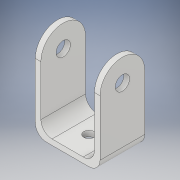
# Autodesk Inventor part: MainMount
Saved by Autodesk Inventor 2018 (Build 220112000, 112)
## iProperties
Created: 2019-05-28
Part Number: MainMount
Material: ABS Plastic
Document SubType Name: Modeling
Designer: Ash
Density: 1.06 g/cm^3
Appearance: Smooth - White
Author: Ash
Autodesk Inventor part; units mm, degrees
ref_plane "YZ Plane" through (0, 0, 0) normal (1, 0, 0) x (0, 1, 0)
ref_plane "XZ Plane" through (0, 0, 0) normal (0, 1, 0) x (-1, 0, 0)
ref_plane "XY Plane" through (0, 0, 0) normal (0, 0, 1) x (1, 0, 0)
sketch "Sketch1" plane through (0, 0, 0) normal (0, 1, 0) x (-1, 0, 0)
  line L0 (0, 0) -> (-30.48, 0)
  line L1 (-30.48, 0) -> (-30.48, -25.4)
  line L2 (-30.48, -25.4) -> (0, -25.4)
  line L3 (0, -25.4) -> (0, 0)
  line L4 (0, -25.4) -> (3.175, -25.4)
  line L5 (3.175, -25.4) -> (3.175, 0)
  line L6 (3.175, 0) -> (0, 0)
  line L7 (0, 0) -> (0, -25.4)
  line L8 (-30.48, -25.4) -> (-33.655, -25.4)
  line L9 (-33.655, -25.4) -> (-33.655, 0)
  line L10 (-33.655, 0) -> (-30.48, 0)
  line L11 (-30.48, 0) -> (-30.48, -25.4)
  dimension "d0" = 30.48
  dimension "d1" = 25.4
  dimension "d2" = 3.175
  dimension "d3" = 3.175
  constraints: 24 end point, 6 parallel, 3 horizontal, 3 perpendicular, 2 collinear
  measures "d0" distance of L2.end L1.end
  measures "d1" distance of L2.end L0.start
  measures "d2" distance of L6.end L5.end
  measures "d3" distance of L9.end L10.end
extrude "Extrusion1" add sketch "Sketch1" along normal blind 3.175 contours L3 L2 L1 L0
extrude "Extrusion2" add sketch "Sketch1" along normal blind 50.8 contours L6 L5 L4 L3 | L1 L8 L9 L10
sketch "Sketch2" plane through (-3.175, 0, -25.4) normal (-1, 0, 0) x (0, 0, 1)
  circle A0 centre (12.7, 38.1) radius 4.064
  line L0 (0, 50.8) -> (25.4, 50.8) projected
  line L1 (12.7, 38.1) -> (0, 38.1) construction
  line L2 (12.7, 38.1) -> (25.4, 38.1) construction
  point P0 (25.4, 0)
  dimension "d8" = 8.128
  dimension "d9" = 12.7
  constraints: 4 end point, 2 horizontal, 1 centre point, 1 collinear
  measures "d8" diameter of A0
  measures "d9" distance from line of L0 L1.start
extrude "Extrusion3" cut sketch "Sketch2" against normal through all
fillet "Fillet1" radius 12.7 4 edges at (-1.5875, 50.8, 0) (32.0675, 50.8, 0) (32.0675, 50.8, -25.4) (-1.5875, 50.8, -25.4)
fillet "Fillet2" radius 6.35 4 edges at (-3.175, 0, -12.7) (0, 3.175, -12.7) (30.48, 3.175, -12.7) (33.655, 0, -12.7)
sketch "Sketch3" plane through (0, 0, 0) normal (0, -1, 0) x (1, 0, 0)
  circle A0 centre (14.605, -12.7) radius 2.921
  line L0 (14.605, -12.7) -> (1.905, -12.7) construction
  line L1 (27.305, 0) -> (27.305, -25.4) construction
  line L2 (3.175, 0) -> (27.305, 0) construction
  line L3 (3.175, -25.4) -> (3.175, 0) construction
  line L4 (27.305, -25.4) -> (3.175, -25.4) construction
  line L5 (14.605, -12.7) -> (27.305, -12.7) construction
  line L6 (14.605, -12.7) -> (14.605, 0) construction
  line L7 (14.605, -12.7) -> (14.605, -25.4) construction
  point P0 (0, 0)
  dimension "d14" = 5.842
  constraints: 8 end point, 3 equal length, 2 point on line, 1 centre point, 1 collinear, 1 horizontal, 1 midpoint, 1 vertical
  measures "d14" diameter of A0
extrude "Extrusion4" cut sketch "Sketch3" against normal through all
body "Solid1"
